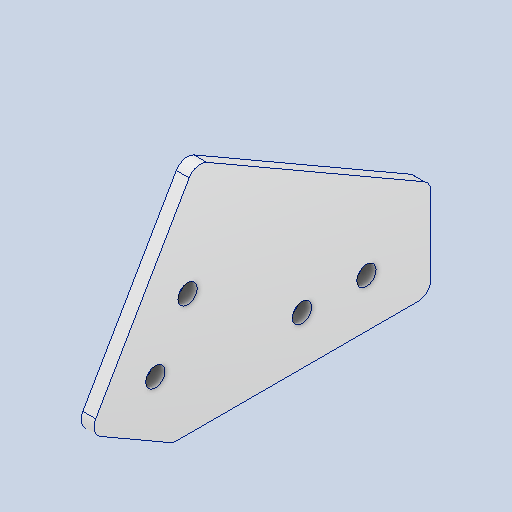
# Autodesk Inventor part: belt_liner_v3_Plate_1
Saved by Autodesk Inventor 2025.2 (Build 292293000, 293)
## iProperties
Created: 2025-01-19
Part Number: belt_liner_v3_Plate_1
Material: アルミニウム 6061
Document SubType Name: Modeling
Designer: haruy
Density: 2.7 g/cm^3
Appearance: アルミニウム - フラット
Author: haruy
Autodesk Inventor part; units mm, degrees
ref_plane "YZ Plane" through (0, 0, 0) normal (1, 0, 0) x (0, 1, 0)
ref_plane "XZ Plane" through (0, 0, 0) normal (0, 1, 0) x (-1, 0, 0)
ref_plane "XY Plane" through (0, 0, 0) normal (0, 0, 1) x (1, 0, 0)
derived "belt_liner_v3_Sketch_Base.ipt"
sketch "スケッチ1" plane through (300, 0, 0) normal (1, 0, 0) x (0, 1, 0)
  circle A0 centre (0, 0) radius 22.36
  circle A1 centre (395.9468, -228.6) radius 23.875 construction
  line L0 (0, 0) -> (0, -985.832)
  line L1 (4.6934, 56.2493) -> (12.1934, 69.2396)
  line L2 (12.1934, 69.2396) -> (479.8471, -200.7604)
  line L3 (479.8471, -200.7604) -> (472.3471, -213.7507)
  line L4 (472.3471, -213.7507) -> (4.6934, 56.2493)
  line L5 (0, 0) -> (395.9468, -228.6)
  line L6 (-43.5991, -27.3958) -> (-51.0991, -40.3862)
  line L7 (-51.0991, -40.3862) -> (364.5498, -280.3612)
  line L8 (364.5498, -280.3612) -> (372.0498, -267.3708)
  line L9 (372.0498, -267.3708) -> (-43.5991, -27.3958)
  line L10 (-64.8558, 113.724) -> (-64.8558, 113.724)
  line L11 (4.6934, 56.2493) -> (0.3513, 58.7562)
  line L12 (0.3513, 58.7562) -> (-2.1487, 54.426)
  line L13 (-2.1487, 54.426) -> (2.1934, 51.9191)
  line L14 (2.1934, 51.9191) -> (4.6934, 56.2493)
  line L15 (472.3471, -213.7507) -> (374.1722, -157.0694)
  line L16 (0, -985.832) -> (0, 0)
  circle A2 centre (0, 0) radius 12.5
  circle A3 centre (0, 0) radius 15
  line L17 (0, 0) -> (0, 0)
  circle A4 centre (0, 0) radius 24.06 construction
  line L18 (0, 0) -> (0, 0)
  line L19 (0, 0) -> (0, 0)
  line L20 (-43.5991, -27.3958) -> (-41.0991, -23.0657)
  line L21 (-41.0991, -23.0657) -> (28.9181, -63.4901)
  line L22 (32.4803, -71.3202) -> (-43.5991, -27.3958)
  line L23 (85.8056, 26.7396) -> (479.8471, -200.7604)
  line L24 (479.8471, -200.7604) -> (482.5971, -195.9972)
  circle A5 centre (395.9468, -228.6) radius 5
  line L25 (372.0498, -267.3708) -> (346.0691, -252.3708)
  line L26 (346.0691, -252.3708) -> (348.5691, -248.0407)
  line L27 (348.5691, -248.0407) -> (374.5498, -263.0407)
  line L28 (374.5498, -263.0407) -> (372.0498, -267.3708)
  circle A6 centre (391.6167, -226.1) radius 5.1
  line L29 (395.9468, -228.6) -> (511.0389, -295.0485)
  circle A7 centre (413.2673, -238.6) radius 5.1
  line L30 (394.1667, -221.6833) -> (415.8173, -234.1833)
  line L31 (389.0667, -230.5167) -> (410.7173, -243.0167)
  circle A8 centre (395.9468, -228.6) radius 22.175 construction
  line L32 (445.9227, -198.4946) -> (429.9227, -226.2074)
  line L33 (429.9227, -226.2074) -> (438.5829, -231.2074)
  line L34 (438.5829, -231.2074) -> (454.5829, -203.4946)
  line L35 (454.5829, -203.4946) -> (445.9227, -198.4946)
  circle A9 centre (391.6167, -226.1) radius 10.1 construction
  circle A10 centre (413.2673, -238.6) radius 10.1 construction
  line L36 (396.6667, -217.3531) -> (418.3173, -229.8531) construction
  line L37 (386.5667, -234.8469) -> (408.2173, -247.3469) construction
  line L38 (396.6667, -217.3531) -> (732.6663, -411.3426) construction
  line L39 (382.8698, -221.05) -> (387.9198, -212.3031) construction
  line L40 (418.3173, -229.8531) -> (773.0938, -434.6834) construction
  line L41 (773.0938, -434.6834) -> (773.431, -434.8781)
  line L42 (0.3513, 58.7562) -> (-2.1487, 54.426)
  line L43 (-2.1487, 54.426) -> (100.4873, -4.8309)
  line L44 (100.4873, -4.8309) -> (102.9873, -0.5007)
  line L45 (102.9873, -0.5007) -> (0.3513, 58.7562)
  line L46 (408.2173, -247.3469) -> (418.3173, -229.8531)
  line L47 (418.3173, -229.8531) -> (426.9776, -234.8531)
  line L48 (426.9776, -234.8531) -> (416.8776, -252.3469)
  line L49 (416.8776, -252.3469) -> (408.2173, -247.3469) construction
  line L50 (479.8471, -200.7604) -> (472.3471, -213.7507)
  line L51 (472.3471, -213.7507) -> (550.2461, -258.7257)
  line L52 (550.2461, -258.7257) -> (557.7461, -245.7353)
  line L53 (557.7461, -245.7353) -> (479.8471, -200.7604)
  line L54 (-12.1522, -2.9282) -> (-38.1087, -47.8862)
  line L55 (-12.1522, -2.9282) -> (25.1838, 61.7396)
  circle A11 centre (38.0844, 34.0842) radius 1.5
  circle A12 centre (59.7351, 21.5842) radius 1.5
  circle A13 centre (364.6396, -260.2057) radius 1.5
  circle A14 centre (0, 0) radius 60
  line L56 (54.6948, -84.1458) -> (57.1948, -79.8157)
  line L57 (100.4873, -4.8309) -> (57.1948, -79.8157)
  circle A15 centre (81.3857, 9.0842) radius 1.5
  circle A16 centre (395.9468, -228.6) radius 6 construction
  circle A17 centre (0, 0) radius 24.06 construction
  circle A18 centre (0, 0) radius 24.06
  circle A19 centre (395.9468, -228.6) radius 24.06
  line L58 (407.9768, -207.7634) -> (12.03, 20.8366)
  circle A20 centre (379.4057, -219.05) radius 4
  circle A21 centre (379.4057, -219.05) radius 1.5
  circle A22 centre (395.9468, -228.6) radius 18.525 construction
  circle A23 centre (402.5334, -217.3917) radius 4
  line L59 (390.9834, -237.3969) -> (396.0334, -228.65)
  circle A24 centre (402.5334, -217.3917) radius 1.5
  line L60 (387.9198, -212.3031) -> (391.3698, -206.3276) construction
  line L61 (391.3698, -206.3276) -> (430.4276, -228.8776)
  line L62 (426.9776, -234.8531) -> (430.4276, -228.8776)
  line L63 (391.3698, -206.3276) -> (377.1969, -215.7152)
  line L64 (374.3698, -235.7724) -> (413.4276, -258.3224)
  line L65 (374.3698, -235.7724) -> (375.4133, -218.8045)
  line L66 (416.8776, -252.3469) -> (413.4276, -258.3224)
  circle A25 centre (389.5334, -239.9083) radius 4
  circle A26 centre (389.5334, -239.9083) radius 1.5
  circle A27 centre (300.5299, 58.6531) radius 120
  line L67 (24.7883, 15.78) -> (16.128, 20.78) construction
  line L68 (550.2461, -258.7257) -> (524.2653, -243.7257)
  line L69 (524.2653, -243.7257) -> (521.7653, -248.0558)
  line L70 (521.7653, -248.0558) -> (547.7461, -263.0558)
  line L71 (547.7461, -263.0558) -> (550.2461, -258.7257)
  circle A28 centre (540.3358, -255.8908) radius 1.5
  line L72 (100.4873, -4.8309) -> (102.9873, -0.5007)
  line L73 (102.9873, -0.5007) -> (112.9466, -6.2507)
  line L74 (112.9466, -6.2507) -> (110.4466, -10.5809)
  line L75 (110.4466, -10.5809) -> (100.4873, -4.8309)
  circle A29 centre (531.6756, -250.8908) radius 1.5
  circle A30 centre (355.9793, -255.2057) radius 1.5
  line L76 (28.9181, -63.4901) -> (57.1948, -79.8157)
  line L77 (479.8471, -200.7604) -> (482.5971, -195.9972)
  line L78 (121.4466, 8.4717) -> (179.9033, -25.2783)
  line L79 (179.9033, -25.2783) -> (182.4033, -20.9482)
  line L80 (182.4033, -20.9482) -> (123.9466, 12.8018)
  line L81 (123.9466, 12.8018) -> (121.4466, 8.4717)
  circle A31 centre (135.9059, 10.5159) radius 4
  circle A32 centre (135.9059, 10.5159) radius 11
  circle A33 centre (161.8867, -4.4841) radius 4
  circle A34 centre (161.8867, -4.4841) radius 11
  line L82 (131.87, -4.4745) -> (128.37, -10.5366)
  line L83 (128.37, -10.5366) -> (147.4226, -21.5366)
  line L84 (147.4226, -21.5366) -> (150.9226, -15.4745)
  line L85 (150.9226, -15.4745) -> (131.87, -4.4745)
  line L86 (141.3963, -9.9745) -> (137.8963, -16.0366)
  line L87 (157.8508, -19.4745) -> (154.3508, -25.5366)
  line L88 (154.3508, -25.5366) -> (173.4033, -36.5366)
  line L89 (173.4033, -36.5366) -> (176.9033, -30.4745)
  line L90 (176.9033, -30.4745) -> (157.8508, -19.4745)
  line L91 (167.377, -24.9745) -> (163.877, -31.0366)
  line L92 (8.4434, 62.7444) -> (553.9961, -252.2305)
  line L93 (170.4033, -41.7328) -> (167.9033, -46.0629)
  line L94 (111.9466, -7.9828) -> (170.4033, -41.7328)
  line L95 (167.9033, -46.0629) -> (109.4466, -12.3129)
  line L96 (109.4466, -12.3129) -> (111.9466, -7.9828)
  circle A35 centre (117.4059, -21.527) radius 11
  circle A36 centre (117.4059, -21.527) radius 4
  circle A37 centre (143.3867, -36.527) radius 11
  circle A38 centre (143.3867, -36.527) radius 4
  line L97 (140.9322, -2.7783) -> (147.8604, -6.7783)
  line L98 (147.8604, -6.7783) -> (138.3604, -23.2328)
  line L99 (138.3604, -23.2328) -> (131.4322, -19.2328)
  line L100 (131.4322, -19.2328) -> (140.9322, -2.7783)
  line L101 (166.9129, -17.7783) -> (173.8411, -21.7783)
  line L102 (173.8411, -21.7783) -> (164.3411, -38.2328)
  line L103 (164.3411, -38.2328) -> (157.4129, -34.2328)
  line L104 (157.4129, -34.2328) -> (166.9129, -17.7783)
  line L105 (109.4466, -12.3129) -> (96.9466, -33.9636)
  line L106 (96.9466, -33.9636) -> (105.6069, -38.9636)
  line L107 (105.6069, -38.9636) -> (118.1069, -17.3129)
  line L108 (118.1069, -17.3129) -> (109.4466, -12.3129)
  line L109 (109.4466, -12.3129) -> (144.9536, -32.8129)
  line L110 (144.9536, -32.8129) -> (140.9536, -39.7411)
  line L111 (140.9536, -39.7411) -> (105.4466, -19.2411)
  line L112 (105.4466, -19.2411) -> (109.4466, -12.3129)
  line L113 (128.9322, -23.5629) -> (135.8604, -27.5629)
  line L114 (135.8604, -27.5629) -> (134.3604, -30.161)
  line L115 (134.3604, -30.161) -> (127.4322, -26.161)
  line L116 (127.4322, -26.161) -> (128.9322, -23.5629)
  circle A39 centre (-7.7081, -45.2307) radius 1.25
  circle A40 centre (13.9426, -57.7307) radius 1.25
  circle A41 centre (35.5932, -70.2307) radius 1.25
  circle A42 centre (300.5299, 58.6531) radius 130
  line L117 (300.5299, 58.6531) -> (196.6069, 118.6531)
  line L118 (300.5299, 58.6531) -> (184.6188, 27.5948)
  line L119 (300.5299, 58.6531) -> (269.4716, 174.5642)
  line L120 (272.4716, 179.7603) -> (181.6188, 22.3986)
  line L121 (181.6188, 22.3986) -> (176.4227, 25.3986)
  line L122 (176.4227, 25.3986) -> (267.2755, 182.7603)
  line L123 (267.2755, 182.7603) -> (272.4716, 179.7603)
  line L124 (300.5299, 58.6531) -> (235.5299, -53.9302)
  line L125 (444.9227, -200.2266) -> (442.4227, -204.5567)
  line L126 (442.4227, -204.5567) -> (500.8794, -238.3067)
  line L127 (500.8794, -238.3067) -> (503.3794, -233.9766)
  line L128 (503.3794, -233.9766) -> (444.9227, -200.2266)
  line L129 (503.3794, -233.9766) -> (500.8794, -238.3067)
  line L130 (500.8794, -238.3067) -> (520.7653, -249.7879)
  line L131 (520.7653, -249.7879) -> (523.2653, -245.4578)
  line L132 (523.2653, -245.4578) -> (503.3794, -233.9766)
  line L133 (391.3698, -206.3276) -> (521.7653, -248.0558)
  circle A43 centre (395.9468, -228.6) radius 34.06
  line L134 (512.7911, -245.184) -> (516.2911, -239.1218)
  circle A44 centre (396.0334, -228.65) radius 8.5
  line L135 (253.2022, 236.6791) -> (109.4466, -12.3129)
  line L136 (249.3989, -49.9085) -> (244.3828, -58.5967)
  line L137 (244.3828, -58.5967) -> (167.9033, -46.0629)
  line L138 (181.6188, 22.3986) -> (198.8709, -5.1077)
  line L139 (267.2755, 182.7603) -> (268.3404, 184.6048)
  circle A45 centre (127.0267, 8.1368) radius 1.5
  circle A46 centre (176.8232, -20.6132) radius 1.5
  circle A47 centre (115.0267, -12.6479) radius 1.5
  circle A48 centre (164.8232, -41.3979) radius 1.5
  line L140 (176.4227, 25.3986) -> (179.4227, 30.5948)
  line L141 (179.4227, 30.5948) -> (175.0925, 33.0948)
  line L142 (175.0925, 33.0948) -> (172.0925, 27.8986)
  line L143 (172.0925, 27.8986) -> (176.4227, 25.3986)
  line L144 (267.2755, 182.7603) -> (264.2755, 177.5642)
  line L145 (264.2755, 177.5642) -> (259.9453, 180.0642)
  line L146 (259.9453, 180.0642) -> (262.9453, 185.2603)
  line L147 (262.9453, 185.2603) -> (267.2755, 182.7603)
  circle A49 centre (263.6104, 181.4122) radius 1.5
  line L148 (268.3404, 184.6048) -> (262.9453, 185.2603)
  line L149 (262.9453, 185.2603) -> (242.1446, 174.8045)
  circle A50 centre (175.7576, 29.2467) radius 1.5
  line L150 (547.7461, -263.0558) -> (372.0498, -267.3708)
  line L151 (348.5691, -248.0407) -> (376.4027, -216.4077)
  line L152 (524.2653, -243.7257) -> (521.7653, -248.0558)
  line L153 (521.7653, -248.0558) -> (514.8371, -244.0558)
  line L154 (514.8371, -244.0558) -> (517.3371, -239.7257)
  line L155 (517.3371, -239.7257) -> (524.2653, -243.7257)
  line L156 (-20.7882, -57.8862) -> (-13.2882, -44.8958)
  line L157 (5.1926, -72.8862) -> (12.6926, -59.8958)
  line L158 (-89.3539, 250.2187) -> (-109.3539, 250.2187)
  line L159 (-109.3539, 250.2187) -> (-109.3539, -699.6003)
  line L160 (-109.3539, -699.6003) -> (-89.3539, -699.6003)
  line L161 (-89.3539, -699.6003) -> (-89.3539, 250.2187)
  line L162 (263.6104, 181.4122) -> (-89.3539, 181.4122)
  circle A51 centre (986.855, -337.5969) radius 120
  line L163 (54.6948, -84.1458) -> (57.1948, -79.8157)
  line L164 (57.1948, -79.8157) -> (67.1541, -85.5657)
  line L165 (67.1541, -85.5657) -> (64.6541, -89.8958)
  line L166 (64.6541, -89.8958) -> (54.6948, -84.1458)
  line L167 (-43.5991, -27.3958) -> (2.1934, 51.9191)
  line L168 (-19.4528, 14.4267) -> (142.0763, -78.8321)
  circle A52 centre (74.6188, -7.5516) radius 15
  line L169 (64.6541, -89.8958) -> (112.9466, -6.2507)
  circle A53 centre (74.6188, -7.5516) radius 22
  circle A54 centre (67.1497, -35.5733) radius 5
  circle A55 centre (103.6165, -12.411) radius 5
  circle A56 centre (65.324, -78.7356) radius 5
  circle A57 centre (11.7598, -74.0723) radius 15
  circle A58 centre (48.162, -57.4928) radius 15
  circle A59 centre (48.162, -57.4928) radius 22
  circle A60 centre (0, 0) radius 24.06
  line L170 (507.8076, -242.3067) -> (511.3076, -236.2446) construction
  line L171 (514.8371, -244.0558) -> (517.3371, -239.7257)
  line L172 (517.3371, -239.7257) -> (511.275, -236.2257)
  line L173 (511.275, -236.2257) -> (508.775, -240.5558)
  line L174 (508.775, -240.5558) -> (514.8371, -244.0558)
  line L175 (-51.0991, -55.3862) -> (-36.0991, -55.3862)
  line L176 (-36.0991, -55.3862) -> (-36.0991, -220.3862)
  line L177 (-36.0991, -220.3862) -> (-51.0991, -220.3862)
  line L178 (-51.0991, -220.3862) -> (-51.0991, -55.3862)
  line L179 (-51.0991, -220.3862) -> (253.9009, -220.3862)
  line L180 (253.9009, -220.3862) -> (253.9009, -235.3862)
  line L181 (253.9009, -235.3862) -> (-51.0991, -235.3862)
  line L182 (-51.0991, -235.3862) -> (-51.0991, -220.3862)
  line L183 (-51.0991, -220.3862) -> (-36.0991, -220.3862)
  line L184 (-36.0991, -220.3862) -> (-36.0991, -235.3862)
  line L185 (-36.0991, -235.3862) -> (-51.0991, -235.3862)
  line L186 (-51.0991, -235.3862) -> (-51.0991, -220.3862)
  line L187 (-51.0991, -40.3862) -> (-51.0991, -55.3862)
  line L188 (-51.0991, -80.3862) -> (-36.0991, -80.3862)
  line L189 (-36.0991, -80.3862) -> (-22.5286, -56.8814)
  line L190 (-22.5286, -56.8814) -> (-15.0286, -43.891)
  circle A61 centre (-32.1936, -42.641) radius 1.5
  circle A62 centre (-40.8539, -37.641) radius 1.5
  circle A63 centre (-43.5991, -60.3862) radius 1.5
  circle A64 centre (-43.5991, -70.3862) radius 1.5
  line L191 (233.9009, -220.3862) -> (233.9009, -235.3862)
  line L192 (253.9009, -220.3862) -> (260.6701, -220.3862)
  line L193 (253.9009, -235.3862) -> (286.6508, -235.3862)
  line L194 (260.6701, -220.3862) -> (268.1701, -207.3958)
  line L195 (286.6508, -235.3862) -> (294.1508, -222.3958)
  circle A65 centre (268.7502, -216.391) radius 1.5
  circle A66 centre (277.4105, -221.391) radius 1.5
  circle A67 centre (248.9009, -227.8862) radius 1.5
  circle A68 centre (238.9009, -227.8862) radius 1.5
  point P0 (732.6663, -411.3426)
  point P1 (-0.8987, 56.5911)
  point P2 (-30.6087, -34.8958)
  point P3 (333.6588, -253.866)
  point P4 (-43.5991, -230.3862)
  point P5 (-43.5991, -220.3862)
  point P6 (-31.0991, -227.8862)
  point P7 (-21.0991, -227.8862)
extrude "押し出し1" add sketch "スケッチ1" against normal blind 2 contours L54 A14 L6 L9 | L9 L190 A14 L54 | A14 L190 L7 L54 | L54 L7 L6 A14 | L7 L189 L176 L175 L187 | L175 L176 L188 L178
fillet "フィレット1" radius 2 5 edges at (299, -36.0991, -80.3862) (299, -51.0991, -80.3862) (299, -51.0991, -40.3862) (299, -43.5991, -27.3958) (299, -15.0286, -43.891)
